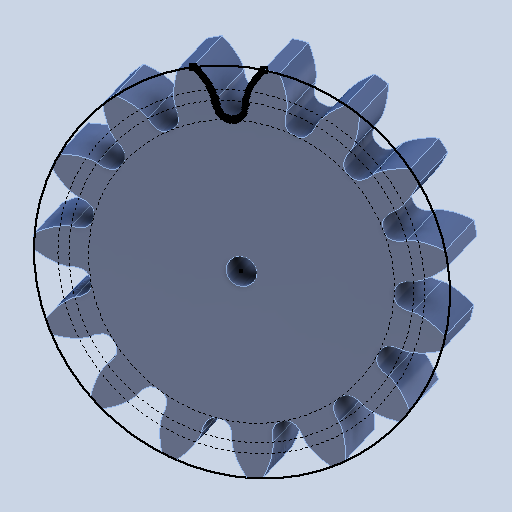
# Autodesk Inventor part: SPUR_06
Saved by Autodesk Inventor 2024 (Build 280153000, 153)
## iProperties
Created: 2023-06-04
Part Number: SPUR_06
Material: Generic
Document SubType Name: Modeling
Designer: Neko-san
Density: 1 g/cm^3
Appearance: Flaked Satin - Blue
Author: Neko-san
Autodesk Inventor part; units mm, degrees
ref_plane "YZ Plane" through (0, 0, 0) normal (1, 0, 0) x (0, 1, 0)
ref_plane "XZ Plane" through (0, 0, 0) normal (0, 1, 0) x (-1, 0, 0)
ref_plane "XY Plane" through (0, 0, 0) normal (0, 0, 1) x (1, 0, 0)
sketch "Sketch1" plane through (0, 0, 0) normal (0, 0, 1) x (1, 0, 0)
  spline S0 degree 3 poles (-5.7795, 33.5052) (-5.6878, 33.4084) (-5.5044, 33.2149) (-5.2376, 32.9168) (-4.9769, 32.6134) (-4.7236, 32.3038) (-4.4778, 31.9882) (-4.2401, 31.6665) (-4.011, 31.3386) (-3.7913, 31.0043) (-3.5815, 30.6637) (-3.3827, 30.3166) (-3.1958, 29.9628) (-3.0224, 29.6023) (-2.8642, 29.2348) (-2.7237, 28.8602) (-2.6258, 28.5414) (-2.561, 28.2826) (-2.5399, 28.1509) (-2.5294, 28.0851) knots 0 0 0 0 0.039997 0.079995 0.119993 0.15999 0.199988 0.239985 0.279982 0.319979 0.359976 0.399973 0.439969 0.479965 0.51996 0.559953 0.599944 0.619941 0.639933 0.639933 0.639933 0.639933
  spline S1 degree 3 poles (-2.5294, 28.0851) (-2.5246, 27.9909) (-2.515, 27.8026) (-2.486, 27.5212) (-2.4404, 27.242) (-2.3816, 26.9652) (-2.3021, 26.6937) (-2.2045, 26.428) (-2.1031, 26.215) (-2.0121, 26.0499) (-1.9106, 25.891) (-1.7978, 25.7394) (-1.6709, 25.5999) (-1.5691, 25.5016) (-1.4617, 25.4096) (-1.3481, 25.3252) (-1.2274, 25.2513) (-1.1038, 25.1826) (-0.9741, 25.1257) (-0.8404, 25.0796) (-0.7043, 25.0406) (-0.5648, 25.0171) (-0.4243, 24.9998) (-0.2356, 24.9979) (0, 25.0014) (0.2356, 24.9979) (0.4243, 24.9998) (0.5648, 25.0171) (0.7043, 25.0406) (0.8404, 25.0796) (0.9741, 25.1257) (1.1038, 25.1826) (1.2274, 25.2513) (1.3481, 25.3252) (1.4617, 25.4096) (1.5691, 25.5016) (1.6709, 25.5999) (1.7978, 25.7394) (1.9106, 25.891) (2.0121, 26.0499) (2.1031, 26.215) (2.2045, 26.428) (2.3021, 26.6937) (2.3816, 26.9652) (2.4404, 27.242) (2.486, 27.5212) (2.515, 27.8026) (2.5246, 27.9909) (2.5294, 28.0851) knots 0 0 0 0 0.028276 0.056553 0.084829 0.113105 0.141379 0.169649 0.197917 0.212055 0.226194 0.254459 0.268599 0.282735 0.296872 0.311012 0.325147 0.339281 0.353421 0.367555 0.381693 0.395831 0.409965 0.424104 0.452382 0.48066 0.494799 0.508933 0.523071 0.537209 0.551343 0.565483 0.579617 0.593752 0.607892 0.622029 0.636165 0.650305 0.67857 0.692709 0.706847 0.735115 0.763385 0.791659 0.819935 0.848211 0.876488 0.904764 0.904764 0.904764 0.904764
  spline S2 degree 3 poles (2.5294, 28.0851) (2.5399, 28.1509) (2.561, 28.2826) (2.6258, 28.5414) (2.7237, 28.8602) (2.8642, 29.2348) (3.0224, 29.6023) (3.1958, 29.9628) (3.3827, 30.3166) (3.5815, 30.6637) (3.7913, 31.0043) (4.011, 31.3386) (4.2401, 31.6665) (4.4778, 31.9882) (4.7236, 32.3038) (4.9769, 32.6134) (5.2376, 32.9168) (5.5044, 33.2149) (5.6878, 33.4084) (5.7795, 33.5052) knots 0 0 0 0 0.019992 0.03999 0.07998 0.119974 0.159969 0.199965 0.239961 0.279957 0.319954 0.359951 0.399948 0.439946 0.479943 0.519941 0.559938 0.599936 0.639933 0.639933 0.639933 0.639933
  circle A0 centre (0, 0) radius 25 construction
  circle A1 centre (0, 0) radius 28.1908 construction
  circle A2 centre (0, 0) radius 30 construction
  circle A3 centre (0, 0) radius 34
  point P0 (-5.5058, 33.2136)
  point P1 (-5.2386, 32.9159)
  point P2 (-4.9781, 32.6124)
  point P3 (-4.7248, 32.3028)
  point P4 (-4.4791, 31.9872)
  point P5 (-4.2415, 31.6655)
  point P6 (-4.0126, 31.3375)
  point P7 (-3.7929, 31.0032)
  point P8 (-3.5833, 30.6626)
  point P9 (-3.3847, 30.3155)
  point P10 (-3.1981, 29.9617)
  point P11 (-3.0249, 29.6011)
  point P12 (-2.8672, 29.2336)
  point P13 (-2.7275, 28.8589)
  point P14 (-2.6107, 28.4764)
  point P15 (-2.5638, 28.282)
  point P16 (-2.5125, 27.8028)
  point P17 (-2.4832, 27.5216)
  point P18 (-2.4382, 27.2424)
  point P19 (-2.3781, 26.9661)
  point P20 (-2.299, 26.6947)
  point P21 (-2.2005, 26.4297)
  point P22 (-2.0796, 26.1742)
  point P23 (-2.0108, 26.0506)
  point P24 (-1.935, 25.9313)
  point P25 (-1.7649, 25.7055)
  point P26 (-1.6698, 25.6009)
  point P27 (-1.5682, 25.5026)
  point P28 (-1.4607, 25.4108)
  point P29 (-1.3469, 25.3269)
  point P30 (-1.2269, 25.2522)
  point P31 (-1.1028, 25.1846)
  point P32 (-0.9734, 25.1275)
  point P33 (-0.84, 25.0808)
  point P34 (-0.7037, 25.0432)
  point P35 (-0.5646, 25.0181)
  point P36 (-0.4241, 25.0025)
  point P37 (-0.2828, 24.9988)
  point P38 (0, 25)
  point P39 (0.2828, 24.9988)
  point P40 (0.4241, 25.0025)
  point P41 (0.5646, 25.0181)
  point P42 (0.7037, 25.0432)
  point P43 (0.84, 25.0808)
  point P44 (0.9734, 25.1275)
  point P45 (1.1028, 25.1846)
  point P46 (1.2269, 25.2522)
  point P47 (1.3469, 25.3269)
  point P48 (1.4607, 25.4108)
  point P49 (1.5682, 25.5026)
  point P50 (1.6698, 25.6009)
  point P51 (1.7649, 25.7055)
  point P52 (1.935, 25.9313)
  point P53 (2.0108, 26.0506)
  point P54 (2.0796, 26.1742)
  point P55 (2.2005, 26.4297)
  point P56 (2.299, 26.6947)
  point P57 (2.3781, 26.9661)
  point P58 (2.4382, 27.2424)
  point P59 (2.4832, 27.5216)
  point P60 (2.5125, 27.8028)
  point P61 (2.5638, 28.282)
  point P62 (2.6107, 28.4764)
  point P63 (2.7275, 28.8589)
  point P64 (2.8672, 29.2336)
  point P65 (3.0249, 29.6011)
  point P66 (3.1981, 29.9617)
  point P67 (3.3847, 30.3155)
  point P68 (3.5833, 30.6626)
  point P69 (3.7929, 31.0032)
  point P70 (4.0126, 31.3375)
  point P71 (4.2415, 31.6655)
  point P72 (4.4791, 31.9872)
  point P73 (4.7248, 32.3028)
  point P74 (4.9781, 32.6124)
  point P75 (5.2386, 32.9159)
  point P76 (5.5058, 33.2136)
  constraints: 4 centre point, 2 point on circle, 169 other
extrude "Extrusion1" add sketch "Sketch1" against normal blind 15
extrude "Extrusion2" cut sketch "Sketch1" against normal through all contours A3 S2 S1 S0 picked at (0.5929, 31.0418)
pattern_circular "Circular Pattern1" count 15 over 360 about axis through (0, 0, 0) along (0, 0, -1) of "Extrusion2"
sketch "Sketch2" plane through (0, 0, 0) normal (0, 0, 1) x (1, 0, 0)
  point P0 (0, 0)
sketch "Sketch3" plane through (0, 0, 0) normal (0, 0, 1) x (1, 0, 0)
  circle A0 centre (0, 0) radius 10
  dimension "d7" = 20
  constraints: 1 centre point, 1 coincident
  measures "d7" diameter of A0
extrude "Extrusion3" cut sketch "Sketch3" against normal through all
sketch "Sketch4" plane through (0, 0, 0) normal (0, 0, 1) x (1, 0, 0)
  point P0 (0, 0)
sketch "Sketch5" plane through (0, 0, -15) normal (0, 0, -1) x (-1, 0, 0)
  circle A0 centre (0, 0) radius 10 projected
  circle A1 centre (0, 0) radius 2.5
  circle A2 centre (0, 0) radius 10
  dimension "d10" = 5
  constraints: 2 centre point, 2 coincident
  measures "d10" diameter of A1
extrude "Extrusion4" add sketch "Sketch5" against normal blind 15
sketch "Sketch6" plane through (0, 0, 0) normal (0, 0, 1) x (1, 0, 0)
  point P0 (0, 0)
equation "\"d0\" = FaceWidth"
equation "\"Module\" = 4"
equation "\"PressureAngle\" = 20deg"
equation "\"UnitProfileClearance\" = 0.25"
equation "\"UnitRoundRadius\" = 0.35"
equation "\"HeadDiameter\" = 68"
equation "\"BaseDiameter\" = 56.38156"
equation "\"FaceWidth\" = 15"
equation "\"HelixAngle\" = 0"
equation "\"UnitCorrection\" = 0"
equation "\"UnitAddendumModification\" = 0"
equation "\"CircularPitch\" = 12.566371"
equation "\"UnitBacklashShift\" = 0"
equation "\"TotalToolShift\" = 0"
equation "\"IsInternal\" = 0"
body "Solid1"
